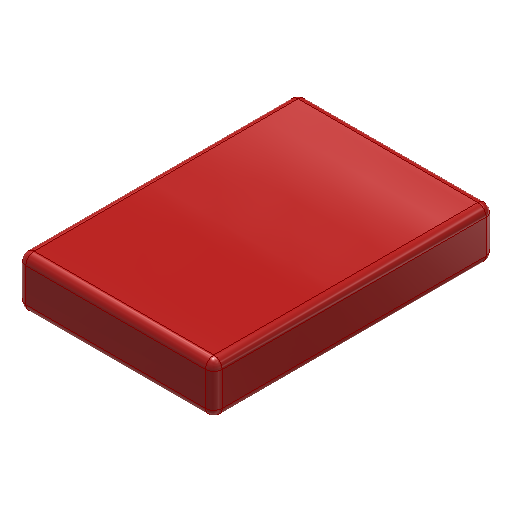
# Autodesk Inventor part: COTS_GENERIC_LiPo_Baterry
Saved by Autodesk Inventor 2025 (Build 290162010, 162A)
## iProperties
Created: 2016-05-01
Part Number: COTS_GENERIC_LiPo_Baterry
Material: Ogólny
Document SubType Name: Modeling
Designer: Andrzej
Density: 1 g/cm^3
Appearance: Czerwona
Mass: 15.573 g
Surface Area: 47.8538 cm^2
Volume: 15.573 cm^3
Author: Andrzej
Autodesk Inventor part; units mm, degrees
ref_plane "YZ Plane" through (0, 0, 0) normal (1, 0, 0) x (0, 1, 0)
ref_plane "XZ Plane" through (0, 0, 0) normal (0, 1, 0) x (-1, 0, 0)
ref_plane "XY Plane" through (0, 0, 0) normal (0, 0, 1) x (1, 0, 0)
sketch "Szkic1" plane through (0, 0, 0) normal (0, 0, 1) x (1, 0, 0)
  line L0 (-3.8809, 1.7985) -> (31.1191, 1.7985)
  line L1 (31.1191, 1.7985) -> (31.1191, -48.2015)
  line L2 (31.1191, -48.2015) -> (-3.8809, -48.2015)
  line L3 (-3.8809, -48.2015) -> (-3.8809, 1.7985)
  point P0 (0, 0)
  dimension "d0" = 35
  dimension "d1" = 50
  constraints: 8 end point, 2 parallel, 1 horizontal, 1 perpendicular
  measures "d0" distance of L1.end L2.end
  measures "d1" distance of L0.end L1.end
extrude "Wyciągnięcie proste1" add sketch "Szkic1" along normal blind 9
fillet "Zaokrąglenie1" radius 1.5 12 edges at (13.6191, 1.7985, 9) (-3.8809, 1.7985, 4.5) (13.6191, 1.7985, 0) (31.1191, 1.7985, 4.5) (31.1191, -23.2015, 9) (-3.8809, -23.2015, 9) (31.1191, -23.2015, 0) (-3.8809, -23.2015, 0) (13.6191, -48.2015, 9) (-3.8809, -48.2015, 4.5) (13.6191, -48.2015, 0) (31.1191, -48.2015, 4.5)
